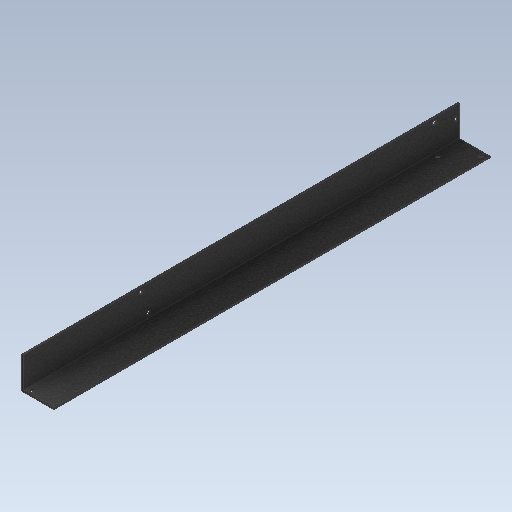
# Autodesk Inventor part: angleline-400
Saved by Autodesk Inventor 2020.4 (Build 244396000, 396)
## iProperties
Created: 2021-02-28
Part Number: angleline-400
Material: Steel
Document SubType Name: Modeling
Designer: AOB
Mass: 481.545 g
Surface Area: 793.702 cm^2
Volume: 61.3433 cm^3
Density: 7.85 g/cm^3
Appearance: Black Cast
Author: AOB
Autodesk Inventor part; units mm, degrees
ref_plane "YZ Plane" through (0, 0, 0) normal (1, 0, 0) x (0, 1, 0)
ref_plane "XZ Plane" through (0, 0, 0) normal (0, 1, 0) x (-1, 0, 0)
ref_plane "XY Plane" through (0, 0, 0) normal (0, 0, 1) x (1, 0, 0)
sketch "Sketch1" plane through (0, 0, 0) normal (0, 0, 1) x (1, 0, 0)
  line L0 (0, 0) -> (0, -38.1)
  line L1 (0, -38.1) -> (38.1, -38.1)
  line L2 (38.1, -38.1) -> (38.1, -36.5125)
  line L3 (38.1, -36.5125) -> (1.5875, -36.5125)
  line L4 (1.5875, -36.5125) -> (1.5875, 0)
  line L5 (1.5875, 0) -> (0, 0)
  dimension "d0" = 1.5875
  dimension "d1" = 1.5875
  dimension "d2" = 38.1
  dimension "d3" = 38.1
  constraints: 12 end point, 5 perpendicular, 1 vertical
  measures "d0" distance of L1.end L2.end
  measures "d1" distance of L4.end L0.start
  measures "d2" distance of L0.start L0.end
  measures "d3" distance of L0.end L1.end
extrude "Extrusion1" add sketch "Sketch1" along normal blind 520
sketch "Sketch2" plane through (0, -38.1, 0) normal (0, -1, 0) x (1, 0, 0)
  line L0 (1.5875, 0.0011) -> (38.1, 0.0011)
  line L1 (38.1, 0.0011) -> (38.1, 36.5136)
  line L2 (38.1, 36.5136) -> (1.5875, 36.5136)
  line L3 (1.5875, 36.5136) -> (1.5875, 0.0011)
  line L4 (1.5875, 483.4864) -> (38.1, 483.4864)
  line L5 (38.1, 483.4864) -> (38.1, 520)
  line L6 (38.1, 520) -> (1.5875, 520)
  line L7 (1.5875, 520) -> (1.5875, 483.4864)
  line L8 (38.1, 37) -> (28.575, 37)
  line L9 (1.5875, 485.3223) -> (1.5875, 520)
  line L10 (0, 0) -> (0, 520) projected
  line L11 (38.1, 483.4864) -> (32.7119, 488.8746)
  line L12 (0, 520) -> (38.1, 520) construction
  line L13 (1.5875, 0) -> (1.5875, 520) construction
  line L14 (0, 0) -> (38.1, 0) construction
  line L15 (1.5875, 520) -> (32.7119, 488.8746)
  line L16 (38.1, 0.0011) -> (1.5875, 36.5136)
  point P0 (6.9757, 31.1254)
  point P1 (6.9756, 514.6118)
  point P2 (32.7124, 5.3887)
  dimension "d6" = 36.5481
  dimension "d12" = 9.525
  dimension "d23" = 7.62
  dimension "d38" = 36.5125
  dimension "d39" = 36.5481
  dimension "d40" = 38.1001
  dimension "d41" = 7.62
  dimension "d81" = 7.62
  dimension "d82" = 7.62
  constraints: 24 end point, 3 horizontal, 3 parallel, 2 point on line, 1 perpendicular, 1 vertical, 5 other
  measures "d6" distance of point (0, 0) L2.end
  measures "d12" distance of L8.start L8.end
  measures "d23" distance of L2.end point (6.976, 31.125)
  measures "d38" distance of L1.end L2.end
  measures "d39" distance of L12.start L4.start
  measures "d40" distance of L12.start L5.end
  measures "d41" distance of L4.end L11.end
  measures "d81" distance of L6.end point (6.976, 514.612)
  measures "d82" distance of point (38.1, 0) point (32.712, 5.389)
hole "Hole1" at (6.9757, -38.1, 31.1254) direction (0, 1, 0) diameter 5 end through all
hole "Hole2" at (32.7119, -38.1, 488.8746) direction (0, 1, 0) diameter 5 end through all
sketch "Sketch3" plane through (0, -38.1, 0) normal (-1, 0, 0) x (0, 0, 1)
  line L0 (0, 38.1) -> (0, 1.5875)
  line L1 (0, 1.5875) -> (34.925, 1.5875)
  line L2 (34.925, 1.5875) -> (34.925, 38.1)
  line L3 (34.925, 38.1) -> (0, 38.1)
  line L4 (365.075, 38.1) -> (365.075, 1.5875)
  line L5 (365.075, 1.5875) -> (401.5875, 1.5875)
  line L6 (401.5875, 1.5875) -> (401.5875, 38.1)
  line L7 (400, 38.1) -> (363.4875, 38.1)
  line L8 (35.4125, 0) -> (35.4125, 9.525)
  line L9 (0, 38.1) -> (37, 38.1)
  line L10 (365.3234, 38.1) -> (400, 38.1)
  line L11 (34.925, 38.1) -> (29.5866, 32.6625)
  line L12 (0, 38.1) -> (400, 38.1)
  line L13 (0, 0) -> (520, 0) construction
  line L14 (3.8007, 1.4875) -> (3.8007, 23.7125) construction
  line L15 (520, 1.5875) -> (520, 38.1) construction
  line L16 (401.5875, 32.6159) -> (379.3625, 32.6159) construction
  line L17 (400, 1.5875) -> (401.5875, 1.5875)
  line L18 (0, 0) -> (0, 1.5875) projected
  line L19 (0, 1.5875) -> (-3.175, 1.5875)
  point P0 (0, 38.1)
  point P1 (520, 38.1)
  point P2 (401.5875, 38.1)
  point P3 (370.4632, 6.9756)
  dimension "d54" = 36.5125
  dimension "d56" = 7.62
  dimension "d76" = 22.225
  dimension "d79" = 1.5875
  constraints: 32 end point, 3 horizontal, 3 parallel, 2 coincident, 2 perpendicular, 2 point on line, 2 vertical, 5 other
  measures "d54" distance of L7.end L7.start
  measures "d56" distance of L4.end point (370.463, 6.976)
  measures "d76" distance of L16.start L16.end
  measures "d79" distance of L17.start L17.end
hole "Hole5" at (0, -31.1244, 370.4632) at (0, -5.4841, 379.3625) at (0, -5.4375, 29.5866) at (0, -14.3875, 3.8007) direction (1, 0, 0) diameter 5 end through all
hole "Hole6" at (6.9756, -38.1, 514.6118) at (32.7124, -38.1, 5.3887) direction (0, 1, 0) diameter 5 end through all
equation "\"d23\" = d14"
equation "\"d54\" = d53"
equation "\"d53\" = 36.5125"
equation "\"d14\" = 7.62"
body "Solid1"
